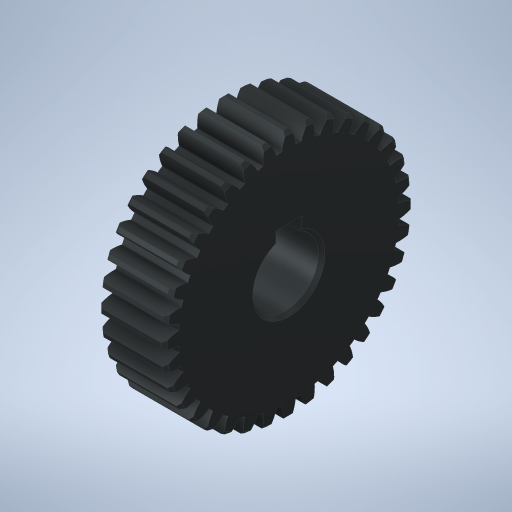
# Autodesk Inventor part: SSA1-36J10_On
Saved by Autodesk Inventor 2023 (Build 270158000, 158)
## iProperties
Category: PARTsolutions
Company: KHK
Created: 2023-07-21
Part Number: SSA1-36J10_On
Material: Iron, Cast
Catalog Web Link: www.cadenas.de
Description: Steel, Hubless Spur Gears (SSA)-
Vendor: KHK
Document SubType Name: Modeling
Designer: psAdmin
Manufacturer: KHK
Mass: 65.5587 g
Surface Area: 44.2777 cm^2
Volume: 9.16905 cm^3
Density: 7.15 g/cm^3
Appearance: Iron Gray
PSOL_IDENT_0: {$CADENAS_DATA/23d-libs/khk/spur_gears/steel_hubless_spur_gears_ssa.prj},198 {VTYP=3D},{NB=SSA1-36J1
PSOL_IDENT_1: 0_On},{LINA=SSA1-36J10},{NN=Steel, Hubless Spur Gears (SSA)},{DATE=06.10.2022 23:14:57},{GEOMDATE=26
PSOL_IDENT_2: .04.2021 06:49:50},{VERSION=},{LINEID=1440},{WBVAR=TOOTH,HT},{WBNUMERIC=}  {NB=SSA1-36J10_On},{LINA=
PSOL_IDENT_3: SSA1-36J10},{KT=DUMMY},{CN=SSA1-36J10},{CN1=SSA1-36J10},{A=10},{VER=1},{KW=4},{KD=1.8},{S=S5K},{SOLD=
PSOL_IDENT_4: S5K},{M=1},{MX=1.000},{Z=36},{B=0},{C=36.0},{D=38.0},{E=10},{F=0},{H=0},{I=0},{WMF=S5001.WMF},{N=0.5
PSOL_IDENT_5: },{L=0.5},{R=0},{L2=0},{VERS=0},{TOOTH=On},{HT=}
NB: SSA1-36J10_On
NN: Steel, Hubless Spur Gears (SSA)
NBSYN: $CN._$TOOTH.
LINA: SSA1-36J10
CATALOG: KHK
CN: SSA1-36J10
A: 10
KW: 4
KD: 1.8
S: S5K
M: 1
Z: 36
C: 36
D: 38
E: 10
TOOTH: On
HT: without
SUPPLIER: KHK
ARTICLENO: SSA1-36J10_On
BOMINFO: SSA1-36J10
CREATOR: CADENAS GmbH
Title: SSA1-36J10
Author: Cadenas PARTsolutions
Autodesk Inventor part; units mm, degrees
ref_plane "YZ Plane" through (0, 0, 0) normal (1, 0, 0) x (0, 1, 0)
ref_plane "XZ Plane" through (0, 0, 0) normal (0, 1, 0) x (-1, 0, 0)
ref_plane "XY Plane" through (0, 0, 0) normal (0, 0, 1) x (1, 0, 0)
sketch "Sketch_1" plane through (0, 0, 0) normal (0, 0, 1) x (1, 0, 0)
  line L0 (10, 0) -> (0, 0)
  line L1 (0, 5.5) -> (0.5, 5)
  line L2 (0.5, 5) -> (9.5, 5)
  line L3 (9.5, 5) -> (10, 5.5)
  line L4 (10, 5.5) -> (10, 18.5)
  line L5 (10, 18.5) -> (9.5, 19)
  line L6 (9.5, 19) -> (0.5, 19)
  line L7 (0.5, 19) -> (0, 18.5)
  line L8 (0, 18.5) -> (0, 5.5)
  constraints: 18 end point
revolve "Revolution1" add sketch "Sketch_1" angle 360 about axis through (10, 0, 0) along (1, 0, 0)
sketch "Sketch_6" plane through (0, 0, 0) normal (1, 0, 0) x (0, 1, 0)
  line L0 (0, 2) -> (0, -2)
  line L1 (0, -2) -> (6.8, -2)
  line L2 (6.8, -2) -> (6.8, 2)
  line L3 (6.8, 2) -> (0, 2)
  constraints: 8 end point
extrude "Extrusion1" cut sketch "Sketch_6" along normal blind 10
sketch "Sketch_7" plane through (0, 0, 0) normal (1, 0, 0) x (0, 1, 0)
  line L0 (38, 38) -> (-38, 38)
  line L1 (-38, 38) -> (-38, -38)
  line L2 (-38, -38) -> (38, -38)
  line L3 (38, -38) -> (38, 38)
  arc A0 (0.3316, 18.9971) -> (-0.3316, 18.9971) centre (0, 0) ccw
  arc A1 (-0.3316, 18.9971) -> (-1.0226, 16.7188) centre (4.9505, 16.1512) ccw
  arc A2 (-1.0226, 16.7188) -> (-1.8962, 16.6423) centre (0, 0) ccw
  arc A3 (-1.8962, 16.6423) -> (-2.9723, 18.7661) centre (-7.68, 15.0462) ccw
  arc A4 (-2.9723, 18.7661) -> (-3.6254, 18.6509) centre (0, 0) ccw
  arc A5 (-3.6254, 18.6509) -> (-3.9102, 16.2872) centre (2.0707, 16.7655) ccw
  arc A6 (-3.9102, 16.2872) -> (-4.7573, 16.0602) centre (0, 0) ccw
  arc A7 (-4.7573, 16.0602) -> (-6.1858, 17.9649) centre (-10.176, 13.484) ccw
  arc A8 (-6.1858, 17.9649) -> (-6.809, 17.738) centre (0, 0) ccw
  arc A9 (-6.809, 17.738) -> (-6.679, 15.3608) centre (-0.8721, 16.8704) ccw
  arc A10 (-6.679, 15.3608) -> (-7.4738, 14.9902) centre (0, 0) ccw
  arc A11 (-7.4738, 14.9902) -> (-9.2114, 16.6178) centre (-12.3629, 11.5121) ccw
  arc A12 (-9.2114, 16.6178) -> (-9.7857, 16.2862) centre (0, 0) ccw
  arc A13 (-9.7857, 16.2862) -> (-9.2449, 13.9676) centre (-3.7883, 16.4626) ccw
  arc A14 (-9.2449, 13.9676) -> (-9.9633, 13.4646) centre (0, 0) ccw
  arc A15 (-9.9633, 13.4646) -> (-11.9571, 14.7658) centre (-14.1741, 9.1904) ccw
  arc A16 (-11.9571, 14.7658) -> (-12.4651, 14.3395) centre (0, 0) ccw
  arc A17 (-12.4651, 14.3395) -> (-11.5299, 12.15) centre (-6.5895, 15.5547) ccw
  arc A18 (-11.5299, 12.15) -> (-12.15, 11.5299) centre (0, 0) ccw
  arc A19 (-12.15, 11.5299) -> (-14.3395, 12.4651) centre (-15.5547, 6.5895) ccw
  arc A20 (-14.3395, 12.4651) -> (-14.7658, 11.9571) centre (0, 0) ccw
  arc A21 (-14.7658, 11.9571) -> (-13.4646, 9.9633) centre (-9.1904, 14.1741) ccw
  arc A22 (-13.4646, 9.9633) -> (-13.9676, 9.2449) centre (0, 0) ccw
  arc A23 (-13.9676, 9.2449) -> (-16.2862, 9.7857) centre (-16.4626, 3.7883) ccw
  arc A24 (-16.2862, 9.7857) -> (-16.6178, 9.2114) centre (0, 0) ccw
  arc A25 (-16.6178, 9.2114) -> (-14.9902, 7.4738) centre (-11.5121, 12.3629) ccw
  arc A26 (-14.9902, 7.4738) -> (-15.3608, 6.679) centre (0, 0) ccw
  arc A27 (-15.3608, 6.679) -> (-17.738, 6.809) centre (-16.8704, 0.8721) ccw
  arc A28 (-17.738, 6.809) -> (-17.9649, 6.1858) centre (0, 0) ccw
  arc A29 (-17.9649, 6.1858) -> (-16.0602, 4.7573) centre (-13.484, 10.176) ccw
  arc A30 (-16.0602, 4.7573) -> (-16.2872, 3.9102) centre (0, 0) ccw
  arc A31 (-16.2872, 3.9102) -> (-18.6509, 3.6254) centre (-16.7655, -2.0707) ccw
  arc A32 (-18.6509, 3.6254) -> (-18.7661, 2.9723) centre (0, 0) ccw
  arc A33 (-18.7661, 2.9723) -> (-16.6423, 1.8962) centre (-15.0462, 7.68) ccw
  arc A34 (-16.6423, 1.8962) -> (-16.7188, 1.0226) centre (0, 0) ccw
  arc A35 (-16.7188, 1.0226) -> (-18.9971, 0.3316) centre (-16.1512, -4.9505) ccw
  arc A36 (-18.9971, 0.3316) -> (-18.9971, -0.3316) centre (0, 0) ccw
  arc A37 (-18.9971, -0.3316) -> (-16.7188, -1.0226) centre (-16.1512, 4.9505) ccw
  arc A38 (-16.7188, -1.0226) -> (-16.6423, -1.8962) centre (0, 0) ccw
  arc A39 (-16.6423, -1.8962) -> (-18.7661, -2.9723) centre (-15.0462, -7.68) ccw
  arc A40 (-18.7661, -2.9723) -> (-18.6509, -3.6254) centre (0, 0) ccw
  arc A41 (-18.6509, -3.6254) -> (-16.2872, -3.9102) centre (-16.7655, 2.0707) ccw
  arc A42 (-16.2872, -3.9102) -> (-16.0602, -4.7573) centre (0, 0) ccw
  arc A43 (-16.0602, -4.7573) -> (-17.9649, -6.1858) centre (-13.484, -10.176) ccw
  arc A44 (-17.9649, -6.1858) -> (-17.738, -6.809) centre (0, 0) ccw
  arc A45 (-17.738, -6.809) -> (-15.3608, -6.679) centre (-16.8704, -0.8721) ccw
  arc A46 (-15.3608, -6.679) -> (-14.9902, -7.4738) centre (0, 0) ccw
  arc A47 (-14.9902, -7.4738) -> (-16.6178, -9.2114) centre (-11.5121, -12.3629) ccw
  arc A48 (-16.6178, -9.2114) -> (-16.2862, -9.7857) centre (0, 0) ccw
  arc A49 (-16.2862, -9.7857) -> (-13.9676, -9.2449) centre (-16.4626, -3.7883) ccw
  arc A50 (-13.9676, -9.2449) -> (-13.4646, -9.9633) centre (0, 0) ccw
  arc A51 (-13.4646, -9.9633) -> (-14.7658, -11.9571) centre (-9.1904, -14.1741) ccw
  arc A52 (-14.7658, -11.9571) -> (-14.3395, -12.4651) centre (0, 0) ccw
  arc A53 (-14.3395, -12.4651) -> (-12.15, -11.5299) centre (-15.5547, -6.5895) ccw
  arc A54 (-12.15, -11.5299) -> (-11.5299, -12.15) centre (0, 0) ccw
  arc A55 (-11.5299, -12.15) -> (-12.4651, -14.3395) centre (-6.5895, -15.5547) ccw
  arc A56 (-12.4651, -14.3395) -> (-11.9571, -14.7658) centre (0, 0) ccw
  arc A57 (-11.9571, -14.7658) -> (-9.9633, -13.4646) centre (-14.1741, -9.1904) ccw
  arc A58 (-9.9633, -13.4646) -> (-9.2449, -13.9676) centre (0, 0) ccw
  arc A59 (-9.2449, -13.9676) -> (-9.7857, -16.2862) centre (-3.7883, -16.4626) ccw
  arc A60 (-9.7857, -16.2862) -> (-9.2114, -16.6178) centre (0, 0) ccw
  arc A61 (-9.2114, -16.6178) -> (-7.4738, -14.9902) centre (-12.3629, -11.5121) ccw
  arc A62 (-7.4738, -14.9902) -> (-6.679, -15.3608) centre (0, 0) ccw
  arc A63 (-6.679, -15.3608) -> (-6.809, -17.738) centre (-0.8721, -16.8704) ccw
  arc A64 (-6.809, -17.738) -> (-6.1858, -17.9649) centre (0, 0) ccw
  arc A65 (-6.1858, -17.9649) -> (-4.7573, -16.0602) centre (-10.176, -13.484) ccw
  arc A66 (-4.7573, -16.0602) -> (-3.9102, -16.2872) centre (0, 0) ccw
  arc A67 (-3.9102, -16.2872) -> (-3.6254, -18.6509) centre (2.0707, -16.7655) ccw
  arc A68 (-3.6254, -18.6509) -> (-2.9723, -18.7661) centre (0, 0) ccw
  arc A69 (-2.9723, -18.7661) -> (-1.8962, -16.6423) centre (-7.68, -15.0462) ccw
  arc A70 (-1.8962, -16.6423) -> (-1.0226, -16.7188) centre (0, 0) ccw
  arc A71 (-1.0226, -16.7188) -> (-0.3316, -18.9971) centre (4.9505, -16.1512) ccw
  arc A72 (-0.3316, -18.9971) -> (0.3316, -18.9971) centre (0, 0) ccw
  arc A73 (0.3316, -18.9971) -> (1.0226, -16.7188) centre (-4.9505, -16.1512) ccw
  arc A74 (1.0226, -16.7188) -> (1.8962, -16.6423) centre (0, 0) ccw
  arc A75 (1.8962, -16.6423) -> (2.9723, -18.7661) centre (7.68, -15.0462) ccw
  arc A76 (2.9723, -18.7661) -> (3.6254, -18.6509) centre (0, 0) ccw
  arc A77 (3.6254, -18.6509) -> (3.9102, -16.2872) centre (-2.0707, -16.7655) ccw
  arc A78 (3.9102, -16.2872) -> (4.7573, -16.0602) centre (0, 0) ccw
  arc A79 (4.7573, -16.0602) -> (6.1858, -17.9649) centre (10.176, -13.484) ccw
  arc A80 (6.1858, -17.9649) -> (6.809, -17.738) centre (0, 0) ccw
  arc A81 (6.809, -17.738) -> (6.679, -15.3608) centre (0.8721, -16.8704) ccw
  arc A82 (6.679, -15.3608) -> (7.4738, -14.9902) centre (0, 0) ccw
  arc A83 (7.4738, -14.9902) -> (9.2114, -16.6178) centre (12.3629, -11.5121) ccw
  arc A84 (9.2114, -16.6178) -> (9.7857, -16.2862) centre (0, 0) ccw
  arc A85 (9.7857, -16.2862) -> (9.2449, -13.9676) centre (3.7883, -16.4626) ccw
  arc A86 (9.2449, -13.9676) -> (9.9633, -13.4646) centre (0, 0) ccw
  arc A87 (9.9633, -13.4646) -> (11.9571, -14.7658) centre (14.1741, -9.1904) ccw
  arc A88 (11.9571, -14.7658) -> (12.4651, -14.3395) centre (0, 0) ccw
  arc A89 (12.4651, -14.3395) -> (11.5299, -12.15) centre (6.5895, -15.5547) ccw
  arc A90 (11.5299, -12.15) -> (12.15, -11.5299) centre (0, 0) ccw
  arc A91 (12.15, -11.5299) -> (14.3395, -12.4651) centre (15.5547, -6.5895) ccw
  arc A92 (14.3395, -12.4651) -> (14.7658, -11.9571) centre (0, 0) ccw
  arc A93 (14.7658, -11.9571) -> (13.4646, -9.9633) centre (9.1904, -14.1741) ccw
  arc A94 (13.4646, -9.9633) -> (13.9676, -9.2449) centre (0, 0) ccw
  arc A95 (13.9676, -9.2449) -> (16.2862, -9.7857) centre (16.4626, -3.7883) ccw
  arc A96 (16.2862, -9.7857) -> (16.6178, -9.2114) centre (0, 0) ccw
  arc A97 (16.6178, -9.2114) -> (14.9902, -7.4738) centre (11.5121, -12.3629) ccw
  arc A98 (14.9902, -7.4738) -> (15.3608, -6.679) centre (0, 0) ccw
  arc A99 (15.3608, -6.679) -> (17.738, -6.809) centre (16.8704, -0.8721) ccw
  arc A100 (17.738, -6.809) -> (17.9649, -6.1858) centre (0, 0) ccw
  arc A101 (17.9649, -6.1858) -> (16.0602, -4.7573) centre (13.484, -10.176) ccw
  arc A102 (16.0602, -4.7573) -> (16.2872, -3.9102) centre (0, 0) ccw
  arc A103 (16.2872, -3.9102) -> (18.6509, -3.6254) centre (16.7655, 2.0707) ccw
  arc A104 (18.6509, -3.6254) -> (18.7661, -2.9723) centre (0, 0) ccw
  arc A105 (18.7661, -2.9723) -> (16.6423, -1.8962) centre (15.0462, -7.68) ccw
  arc A106 (16.6423, -1.8962) -> (16.7188, -1.0226) centre (0, 0) ccw
  arc A107 (16.7188, -1.0226) -> (18.9971, -0.3316) centre (16.1512, 4.9505) ccw
  arc A108 (18.9971, -0.3316) -> (18.9971, 0.3316) centre (0, 0) ccw
  arc A109 (18.9971, 0.3316) -> (16.7188, 1.0226) centre (16.1512, -4.9505) ccw
  arc A110 (16.7188, 1.0226) -> (16.6423, 1.8962) centre (0, 0) ccw
  arc A111 (16.6423, 1.8962) -> (18.7661, 2.9723) centre (15.0462, 7.68) ccw
  arc A112 (18.7661, 2.9723) -> (18.6509, 3.6254) centre (0, 0) ccw
  arc A113 (18.6509, 3.6254) -> (16.2872, 3.9102) centre (16.7655, -2.0707) ccw
  arc A114 (16.2872, 3.9102) -> (16.0602, 4.7573) centre (0, 0) ccw
  arc A115 (16.0602, 4.7573) -> (17.9649, 6.1858) centre (13.484, 10.176) ccw
  arc A116 (17.9649, 6.1858) -> (17.738, 6.809) centre (0, 0) ccw
  arc A117 (17.738, 6.809) -> (15.3608, 6.679) centre (16.8704, 0.8721) ccw
  arc A118 (15.3608, 6.679) -> (14.9902, 7.4738) centre (0, 0) ccw
  arc A119 (14.9902, 7.4738) -> (16.6178, 9.2114) centre (11.5121, 12.3629) ccw
  arc A120 (16.6178, 9.2114) -> (16.2862, 9.7857) centre (0, 0) ccw
  arc A121 (16.2862, 9.7857) -> (13.9676, 9.2449) centre (16.4626, 3.7883) ccw
  arc A122 (13.9676, 9.2449) -> (13.4646, 9.9633) centre (0, 0) ccw
  arc A123 (13.4646, 9.9633) -> (14.7658, 11.9571) centre (9.1904, 14.1741) ccw
  arc A124 (14.7658, 11.9571) -> (14.3395, 12.4651) centre (0, 0) ccw
  arc A125 (14.3395, 12.4651) -> (12.15, 11.5299) centre (15.5547, 6.5895) ccw
  arc A126 (12.15, 11.5299) -> (11.5299, 12.15) centre (0, 0) ccw
  arc A127 (11.5299, 12.15) -> (12.4651, 14.3395) centre (6.5895, 15.5547) ccw
  arc A128 (12.4651, 14.3395) -> (11.9571, 14.7658) centre (0, 0) ccw
  arc A129 (11.9571, 14.7658) -> (9.9633, 13.4646) centre (14.1741, 9.1904) ccw
  arc A130 (9.9633, 13.4646) -> (9.2449, 13.9676) centre (0, 0) ccw
  arc A131 (9.2449, 13.9676) -> (9.7857, 16.2862) centre (3.7883, 16.4626) ccw
  arc A132 (9.7857, 16.2862) -> (9.2114, 16.6178) centre (0, 0) ccw
  arc A133 (9.2114, 16.6178) -> (7.4738, 14.9902) centre (12.3629, 11.5121) ccw
  arc A134 (7.4738, 14.9902) -> (6.679, 15.3608) centre (0, 0) ccw
  arc A135 (6.679, 15.3608) -> (6.809, 17.738) centre (0.8721, 16.8704) ccw
  arc A136 (6.809, 17.738) -> (6.1858, 17.9649) centre (0, 0) ccw
  arc A137 (6.1858, 17.9649) -> (4.7573, 16.0602) centre (10.176, 13.484) ccw
  arc A138 (4.7573, 16.0602) -> (3.9102, 16.2872) centre (0, 0) ccw
  arc A139 (3.9102, 16.2872) -> (3.6254, 18.6509) centre (-2.0707, 16.7655) ccw
  arc A140 (3.6254, 18.6509) -> (2.9723, 18.7661) centre (0, 0) ccw
  arc A141 (2.9723, 18.7661) -> (1.8962, 16.6423) centre (7.68, 15.0462) ccw
  arc A142 (1.8962, 16.6423) -> (1.0226, 16.7188) centre (0, 0) ccw
  arc A143 (1.0226, 16.7188) -> (0.3316, 18.9971) centre (-4.9505, 16.1512) ccw
  constraints: 288 point on circle, 144 centre point, 8 end point
extrude "Extrusion2" cut sketch "Sketch_7" along normal blind 10
body "Solid1"
